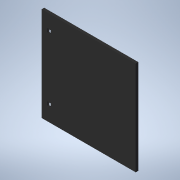
# Autodesk Inventor part: 166X_01_01(2)_P2
Saved by Autodesk Inventor 2021 (Build 250183000, 183)
## iProperties
Created: 2025-08-26
Part Number: 166X_01_01(2)_P2
Material: Generic
Catalog Web Link: www.cadenas.de
Description: AE 2.0 Einzeltuer-AE 2.0 Einzeltuer
Vendor: RITTAL
Document SubType Name: Modeling
Designer: psAdmin
Manufacturer: RITTAL
Mass: 775.853 g
Surface Area: 8964.35 cm^2
Volume: 775.853 cm^3
Density: 1 g/cm^3
Appearance: PSOLRGB-176-176-176
Category: PARTsolutions
Company: RITTAL
Title: 166X_01_01(2)_P2
Author: Cadenas PARTsolutions
Comments: AE 2.0 Einzeltuer
PSOL_IDENT_0: {$CADENAS_DATA/23d-libs/rittal/schaltschranksys/kompakt_schaltschr/parts_ae_2_0/einzeltuer_ae_2_0.pr
PSOL_IDENT_1: j},196 {VTYP=3D},{NB=166X_01_01(2)_P2},{LINA=166X_01_01(2)_P2},{NN=AE 2.0 Einzeltuer},{DATE=28.04.20
PSOL_IDENT_2: 25 21:11:31},{GEOMDATE=11.04.2025 11:21:47},{VERSION=},{LINEID=350},{WBVAR=DETAIL},{WBNUMERIC=DETAIL
PSOL_IDENT_3: }  {NB=166X_01_01(2)_P2},{LINA=166X_01_01(2)_P2},{KT=DUMMY},{BEST=166X},{DETAIL=2},{BEZ1=Neues Kompa
PSOL_IDENT_4: ktgehäuse},{BEZ2=Stahlblech},{BEZ3=eintürig},{B=600},{H=600},{VERS=1},{W=594},{W1=525},{W3=0},{HH=59
PSOL_IDENT_5: 4},{H1=475},{H2=540},{H4=58.0},{H5=400.000},{H6=450.000},{H7=450.000},{D=16.5},{ST=1.5},{R1=5.0},{GE
PSOL_IDENT_6: W=0},{CNSECLASS51=27-18-01-02},{CNSECLASS70=27-18-01-01},{CNSECLASS80=27-18-01-01},{CNSETIM40=EC0002
PSOL_IDENT_7: 61}
NB: 166X_01_01(2)_P2
NN: AE 2.0 Einzeltuer
NT: AE 2.0 Einzeltuer
NBSYN: $BEST._01_01($DETAIL.)_P2
LINA: 166X_01_01(2)_P2
CATALOG: Rittal
BEST: 166X
DETAIL: niedrig
BEZ1: Neues Kompaktgehäuse
BEZ2: Stahlblech
BEZ3: eintürig
B: 600
H: 600
VERS: 1
W: 594
W1: 525
W3: 0
HH: 594
H1: 475
H2: 540
H4: 58
H5: 400
H6: 450
H7: 450
D: 16.5
ST: 1.5
R1: 5
GEW: 0
CNSECLASS70: 27-18-01-01
CNSECLASS80: 27-18-01-01
SUPPLIER: RITTAL
ARTICLENO: 166X_01_01(2)_P2
BOMINFO: 166X_01_01(2)_P2
CREATOR: CADENAS GmbH
Autodesk Inventor part; units mm, degrees
sketch "Sketch_1" plane through (0, 0, 0) normal (0, 1, 0) x (1, 0, 0)
  line L0 (-297, 16.5) -> (-297, 0)
  line L1 (-297, 0) -> (297, 0)
  line L2 (297, 0) -> (297, 16.5)
  line L3 (297, 16.5) -> (295.5, 16.5)
  line L4 (295.5, 16.5) -> (295.5, 1.5)
  line L5 (295.5, 1.5) -> (-295.5, 1.5)
  line L6 (-295.5, 1.5) -> (-295.5, 16.5)
  line L7 (-295.5, 16.5) -> (-297, 16.5)
  constraints: 16 end point
extrude "Extrusion1" add sketch "Sketch_1" along normal mid plane 594
sketch "Sketch_2" plane through (0, 0, 0) normal (1, 0, 0) x (0, 0, -1)
  line L0 (0, -297) -> (16.5, -297)
  line L1 (16.5, -297) -> (16.5, -295.5)
  line L2 (16.5, -295.5) -> (1.5, -295.5)
  line L3 (1.5, -295.5) -> (1.5, 295.5)
  line L4 (1.5, 295.5) -> (16.5, 295.5)
  line L5 (16.5, 295.5) -> (16.5, 297)
  line L6 (16.5, 297) -> (0, 297)
  line L7 (0, 297) -> (0, -297)
  constraints: 16 end point
extrude "Extrusion2" add sketch "Sketch_2" along normal mid plane 594
sketch "Sketch_49" plane through (-291, 274.6934, 0) normal (-0.6389711, 0.7692308, 0) x (0.7692308, 0.6389711, 0)
  line L0 (13, 6.6962) -> (13, 1.5)
  line L1 (13, 1.5) -> (4, 1.5)
  arc A0 (13, 6.6962) -> (4, 1.5) centre (10, 1.5) ccw
  line L2 (13, 6.6962) -> (13, 1.5)
  constraints: 6 end point, 2 point on circle, 1 centre point
revolve "Revolution1" add sketch "Sketch_49" angle 169.43 about axis through (-281, 283, -6.6962) along (0, 0, -1)
sketch "Sketch_7" plane through (0, -237.5, 0) normal (0, 1, 0) x (1, 0, 0)
  arc A0 (290.5, 14.6) -> (290.5, 6.4) centre (290.5, 10.5) ccw
  line L0 (290.5, 6.4) -> (295.5, 6.4)
  line L1 (295.5, 6.4) -> (295.5, 7.9)
  line L2 (295.5, 7.9) -> (290.5, 7.9)
  arc A1 (290.5, 13.1) -> (290.5, 7.9) centre (290.5, 10.5) ccw
  line L3 (290.5, 13.1) -> (295.5, 13.1)
  line L4 (295.5, 13.1) -> (295.5, 14.6)
  line L5 (295.5, 14.6) -> (290.5, 14.6)
  constraints: 12 end point, 4 point on circle, 2 centre point
extrude "Extrusion3" add sketch "Sketch_7" along normal mid plane 19.7
sketch "Sketch_8" plane through (0, 237.5, 0) normal (0, 1, 0) x (1, 0, 0)
  arc A0 (290.5, 14.6) -> (290.5, 6.4) centre (290.5, 10.5) ccw
  line L0 (290.5, 6.4) -> (295.5, 6.4)
  line L1 (295.5, 6.4) -> (295.5, 7.9)
  line L2 (295.5, 7.9) -> (290.5, 7.9)
  arc A1 (290.5, 13.1) -> (290.5, 7.9) centre (290.5, 10.5) ccw
  line L3 (290.5, 13.1) -> (295.5, 13.1)
  line L4 (295.5, 13.1) -> (295.5, 14.6)
  line L5 (295.5, 14.6) -> (290.5, 14.6)
  constraints: 12 end point, 4 point on circle, 2 centre point
extrude "Extrusion4" add sketch "Sketch_8" along normal mid plane 19.7
sketch "Sketch_11" plane through (0, 0, 0) normal (0, 1, 0) x (1, 0, 0)
  line L0 (254.5, 17) -> (254.5, 1.5)
  line L1 (254.5, 1.5) -> (255.3, 1.5)
  line L2 (255.3, 1.5) -> (255.3, 16.2)
  line L3 (255.3, 16.2) -> (269.2, 16.2)
  line L4 (269.2, 16.2) -> (269.2, 1.5)
  line L5 (269.2, 1.5) -> (270, 1.5)
  line L6 (270, 1.5) -> (270, 17)
  line L7 (270, 17) -> (254.5, 17)
  constraints: 16 end point
extrude "Extrusion5" add sketch "Sketch_11" along normal mid plane 540
sketch "Sketch_12" plane through (0, 0, 0) normal (0, 1, 0) x (1, 0, 0)
  line L0 (-270.5, 17) -> (-270.5, 1.5)
  line L1 (-270.5, 1.5) -> (-269.7, 1.5)
  line L2 (-269.7, 1.5) -> (-269.7, 16.2)
  line L3 (-269.7, 16.2) -> (-255.8, 16.2)
  line L4 (-255.8, 16.2) -> (-255.8, 1.5)
  line L5 (-255.8, 1.5) -> (-255, 1.5)
  line L6 (-255, 1.5) -> (-255, 17)
  line L7 (-255, 17) -> (-270.5, 17)
  constraints: 16 end point
extrude "Extrusion6" add sketch "Sketch_12" along normal mid plane 540
sketch "Sketch_13" plane through (262.25, 0, 0) normal (1, 0, 0) x (0, 0, -1)
  line L0 (14, 239.5) -> (18, 239.5)
  line L1 (18, 239.5) -> (18, -239.5)
  line L2 (18, -239.5) -> (14, -239.5)
  line L3 (14, -239.5) -> (14, -252)
  line L4 (14, -252) -> (22, -252)
  line L5 (22, -252) -> (22, 252)
  line L6 (22, 252) -> (14, 252)
  line L7 (14, 252) -> (14, 239.5)
  constraints: 16 end point
extrude "Extrusion7" cut sketch "Sketch_13" along normal mid plane 15.5
sketch "Sketch_14" plane through (-262.75, 0, 0) normal (1, 0, 0) x (0, 0, -1)
  line L0 (14, 239.5) -> (18, 239.5)
  line L1 (18, 239.5) -> (18, -239.5)
  line L2 (18, -239.5) -> (14, -239.5)
  line L3 (14, -239.5) -> (14, -252)
  line L4 (14, -252) -> (22, -252)
  line L5 (22, -252) -> (22, 252)
  line L6 (22, 252) -> (14, 252)
  line L7 (14, 252) -> (14, 239.5)
  constraints: 16 end point
extrude "Extrusion8" cut sketch "Sketch_14" along normal mid plane 15.5
sketch "Sketch_60" plane through (0, 0, -1.5) normal (0, 0, 1) x (1, 0, 0)
  line L0 (-290, -279.7496) -> (-290, -286.7279)
  line L1 (-290, -286.7279) -> (-284.7279, -292)
  line L2 (-284.7279, -292) -> (-277.7496, -292)
  line L3 (-277.7496, -292) -> (-274.138, -289)
  line L4 (-274.138, -289) -> (274.138, -289)
  line L5 (274.138, -289) -> (277.7496, -292)
  line L6 (277.7496, -292) -> (284.7279, -292)
  line L7 (284.7279, -292) -> (290, -286.7279)
  line L8 (290, -286.7279) -> (290, -279.7496)
  line L9 (290, -279.7496) -> (287.0449, -276.192)
  line L10 (287.0449, -276.192) -> (286.5, -258)
  line L11 (286.5, -258) -> (286.5, 258)
  line L12 (286.5, 258) -> (287.0449, 276.192)
  line L13 (287.0449, 276.192) -> (290, 279.7496)
  line L14 (290, 279.7496) -> (290, 286.7279)
  line L15 (290, 286.7279) -> (284.7279, 292)
  line L16 (284.7279, 292) -> (277.7496, 292)
  line L17 (277.7496, 292) -> (274.138, 289)
  line L18 (274.138, 289) -> (-274.138, 289)
  line L19 (-274.138, 289) -> (-277.7496, 292)
  line L20 (-277.7496, 292) -> (-284.7279, 292)
  line L21 (-284.7279, 292) -> (-290, 286.7279)
  line L22 (-290, 286.7279) -> (-290, 279.7496)
  line L23 (-290, 279.7496) -> (-287.0449, 276.192)
  line L24 (-287.0449, 276.192) -> (-286.5, 258)
  line L25 (-286.5, 258) -> (-286.5, -258)
  line L26 (-286.5, -258) -> (-287.0449, -276.192)
  line L27 (-287.0449, -276.192) -> (-290, -279.7496)
  line L28 (-275.5, -258) -> (-274.9551, -276.192)
  line L29 (-274.9551, -276.192) -> (-274.284, -277)
  line L30 (-274.284, -277) -> (274.284, -277)
  line L31 (274.284, -277) -> (274.9551, -276.192)
  line L32 (274.9551, -276.192) -> (275.5, -258)
  line L33 (275.5, -258) -> (275.5, 258)
  line L34 (275.5, 258) -> (274.9551, 276.192)
  line L35 (274.9551, 276.192) -> (274.284, 277)
  line L36 (274.284, 277) -> (-274.284, 277)
  line L37 (-274.284, 277) -> (-274.9551, 276.192)
  line L38 (-274.9551, 276.192) -> (-275.5, 258)
  line L39 (-275.5, 258) -> (-275.5, -258)
  constraints: 80 end point
extrude "Extrusion9" add sketch "Sketch_60" against normal blind 6
sketch "Sketch_27" plane through (0, 0, -17) normal (0, 0, 1) x (1, 0, 0)
  line L0 (-265.6, 180) -> (-250.6, 180)
  line L1 (-250.6, 180) -> (-250.6, 220)
  line L2 (-250.6, 220) -> (-265.6, 220)
  line L3 (-265.6, 220) -> (-265.6, 180)
  constraints: 8 end point
extrude "Extrusion10" cut sketch "Sketch_27" along normal blind 15.5
sketch "Sketch_28" plane through (0, 0, -17) normal (0, 0, 1) x (1, 0, 0)
  line L0 (-265.6, -220) -> (-250.6, -220)
  line L1 (-250.6, -220) -> (-250.6, -180)
  line L2 (-250.6, -180) -> (-265.6, -180)
  line L3 (-265.6, -180) -> (-265.6, -220)
  constraints: 8 end point
extrude "Extrusion11" cut sketch "Sketch_28" along normal blind 15.5
sketch "Sketch_29" plane through (0, 0, -17) normal (0, 0, 1) x (1, 0, 0)
  line L0 (257, 252) -> (257, 251)
  line L1 (257, 251) -> (267.5, 251)
  line L2 (267.5, 251) -> (267.5, 252)
  line L3 (267.5, 252) -> (266.5, 252)
  line L4 (266.5, 252) -> (266.5, 260.5)
  arc A0 (266.5, 260.5) -> (258, 260.5) centre (262.25, 260.5) ccw
  line L5 (258, 260.5) -> (258, 252)
  line L6 (258, 252) -> (257, 252)
  constraints: 14 end point, 2 point on circle, 1 centre point
extrude "Extrusion12" cut sketch "Sketch_29" along normal blind 0.8
sketch "Sketch_30" plane through (0, 0, -17) normal (0, 0, 1) x (1, 0, 0)
  line L0 (257, -252) -> (258, -252)
  line L1 (258, -252) -> (258, -260.5)
  arc A0 (258, -260.5) -> (266.5, -260.5) centre (262.25, -260.5) ccw
  line L2 (266.5, -260.5) -> (266.5, -252)
  line L3 (266.5, -252) -> (267.5, -252)
  line L4 (267.5, -252) -> (267.5, -251)
  line L5 (267.5, -251) -> (257, -251)
  line L6 (257, -251) -> (257, -252)
  constraints: 14 end point, 2 point on circle, 1 centre point
extrude "Extrusion13" cut sketch "Sketch_30" along normal blind 0.8
sketch "Sketch_31" plane through (0, 0, -17) normal (0, 0, 1) x (1, 0, 0)
  line L0 (-268, 252) -> (-268, 251)
  line L1 (-268, 251) -> (-257.5, 251)
  line L2 (-257.5, 251) -> (-257.5, 252)
  line L3 (-257.5, 252) -> (-258.5, 252)
  line L4 (-258.5, 252) -> (-258.5, 260.5)
  arc A0 (-258.5, 260.5) -> (-267, 260.5) centre (-262.75, 260.5) ccw
  line L5 (-267, 260.5) -> (-267, 252)
  line L6 (-267, 252) -> (-268, 252)
  constraints: 14 end point, 2 point on circle, 1 centre point
extrude "Extrusion14" cut sketch "Sketch_31" along normal blind 0.8
sketch "Sketch_32" plane through (0, 0, -17) normal (0, 0, 1) x (1, 0, 0)
  line L0 (-268, -252) -> (-267, -252)
  line L1 (-267, -252) -> (-267, -260.5)
  arc A0 (-267, -260.5) -> (-258.5, -260.5) centre (-262.75, -260.5) ccw
  line L2 (-258.5, -260.5) -> (-258.5, -252)
  line L3 (-258.5, -252) -> (-257.5, -252)
  line L4 (-257.5, -252) -> (-257.5, -251)
  line L5 (-257.5, -251) -> (-268, -251)
  line L6 (-268, -251) -> (-268, -252)
  constraints: 14 end point, 2 point on circle, 1 centre point
extrude "Extrusion15" cut sketch "Sketch_32" along normal blind 0.8
sketch "Sketch_33" plane through (0, 0, 0) normal (0, 0, 1) x (1, 0, 0)
  line L0 (-261.15, 188.85) -> (-238.85, 188.85)
  line L1 (-238.85, 188.85) -> (-238.85, 211.15)
  line L2 (-238.85, 211.15) -> (-253.15, 211.15)
  line L3 (-253.15, 211.15) -> (-253.15, 212.65)
  line L4 (-253.15, 212.65) -> (-259.15, 212.65)
  line L5 (-259.15, 212.65) -> (-259.15, 211.15)
  line L6 (-259.15, 211.15) -> (-261.15, 211.15)
  line L7 (-261.15, 211.15) -> (-261.15, 188.85)
  constraints: 16 end point
extrude "Extrusion16" cut sketch "Sketch_33" against normal blind 1.5
sketch "Sketch_34" plane through (0, 0, 0) normal (0, 0, 1) x (1, 0, 0)
  line L0 (-261.15, -211.15) -> (-238.85, -211.15)
  line L1 (-238.85, -211.15) -> (-238.85, -188.85)
  line L2 (-238.85, -188.85) -> (-253.15, -188.85)
  line L3 (-253.15, -188.85) -> (-253.15, -187.35)
  line L4 (-253.15, -187.35) -> (-259.15, -187.35)
  line L5 (-259.15, -187.35) -> (-259.15, -188.85)
  line L6 (-259.15, -188.85) -> (-261.15, -188.85)
  line L7 (-261.15, -188.85) -> (-261.15, -211.15)
  constraints: 16 end point
extrude "Extrusion17" cut sketch "Sketch_34" against normal blind 1.5
ref_plane "ET_XY" through (290.5, -237.5, -10.5) normal (0, 1, 0) x (1, 0, 0)
ref_plane "ET_YZ" through (290.5, -237.5, -10.5) normal (1, 0, 0) x (0, 0, -1)
ref_plane "ET_ZX" through (290.5, -237.5, -10.5) normal (0, 0, -1) x (0, 1, 0)
ref_plane "SC_XY" through (295.5, 0, 0) normal (0, 0, -1) x (1, 0, 0)
ref_plane "SC_YZ" through (295.5, 0, 0) normal (1, 0, 0) x (0, -1, 0)
ref_plane "SC_ZX" through (295.5, 0, 0) normal (0, -1, 0) x (0, 0, -1)
ref_plane "VV1_XY" through (-250, 200, 0) normal (0, 0, -1) x (1, 0, 0)
ref_plane "VV1_YZ" through (-250, 200, 0) normal (1, 0, 0) x (0, -1, 0)
ref_plane "VV1_ZX" through (-250, 200, 0) normal (0, -1, 0) x (0, 0, -1)
ref_plane "VV2_XY" through (-250, -200, 0) normal (0, 0, -1) x (1, 0, 0)
ref_plane "VV2_YZ" through (-250, -200, 0) normal (1, 0, 0) x (0, -1, 0)
ref_plane "VV2_ZX" through (-250, -200, 0) normal (0, -1, 0) x (0, 0, -1)
ref_plane "to_Auflaufelement_XY" through (-262.75, -260.5, -17) normal (0, 0, 1) x (1, 0, 0)
ref_plane "to_Auflaufelement_YZ" through (-262.75, -260.5, -17) normal (1, 0, 0) x (0, 1, 0)
ref_plane "to_Auflaufelement_ZX" through (-262.75, -260.5, -17) normal (0, 1, 0) x (0, 0, 1)
body "Solid1"
